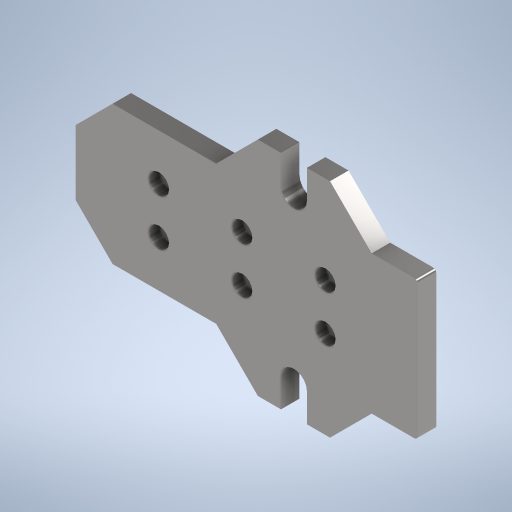
# Autodesk Inventor part: Grundplate
Saved by Autodesk Inventor 2023.2 (Build 272271000, 271)
## iProperties
Created: 2023-02-02
Part Number: Grundplate
Material: Steel, Mild
Document SubType Name: Modeling
Designer: Aditya
Density: 7.85 g/cm^3
Appearance: Semi-Polished
Author: Aditya
Autodesk Inventor part; units mm, degrees
ref_plane "YZ Plane" through (0, 0, 0) normal (1, 0, 0) x (0, 1, 0)
ref_plane "XZ Plane" through (0, 0, 0) normal (0, 1, 0) x (-1, 0, 0)
ref_plane "XY Plane" through (0, 0, 0) normal (0, 0, 1) x (1, 0, 0)
sketch "Sketch1" plane through (0, 0, 0) normal (0, 0, 1) x (1, 0, 0)
  line L0 (92.5, -35.5) -> (92.5, 35.5)
  line L1 (-92.5, 17.5) -> (-92.5, -17.5)
  line L2 (-92.5, 0) -> (-92.5, 17.5)
  line L3 (-92.5, 17.5) -> (-72.5, 37.5)
  line L4 (-92.5, 17.5) -> (-35.0841, 17.5) construction
  line L5 (-92.5, 0) -> (-92.5, -17.5)
  line L6 (-92.5, -17.5) -> (-72.5, -37.5)
  line L7 (25.5, 37.5) -> (25.5, 44.5)
  arc A0 (18.5, 44.5) -> (32.5, 44.5) centre (25.5, 44.5) ccw
  line L8 (32.5, 44.5) -> (32.5, 60)
  line L9 (18.5, 44.5) -> (18.5, 60)
  line L10 (32.5, 60) -> (45, 60)
  line L11 (45, 60) -> (67.5, 37.5)
  line L12 (45, 60) -> (96.9057, 60) construction
  line L13 (18.5, 60) -> (6, 60)
  line L14 (6, 60) -> (-16.5, 37.5)
  line L15 (90.5, 37.5) -> (67.5, 37.5)
  line L16 (-16.5, 37.5) -> (-72.5, 37.5)
  line L17 (25.5, -37.5) -> (25.5, -44.5)
  arc A1 (32.5, -44.5) -> (18.5, -44.5) centre (25.5, -44.5) ccw
  line L18 (18.5, -44.5) -> (18.5, -60)
  line L19 (32.5, -44.5) -> (32.5, -60)
  line L20 (18.5, -60) -> (6, -60)
  line L21 (6, -60) -> (-16.5, -37.5)
  line L22 (32.5, -60) -> (45, -60)
  line L23 (45, -60) -> (67.5, -37.5)
  line L24 (-72.5, -37.5) -> (-16.5, -37.5)
  line L25 (67.5, -37.5) -> (90.5, -37.5)
  arc A2 (92.5, 35.5) -> (90.5, 37.5) centre (90.5, 35.5) ccw
  arc A3 (90.5, -37.5) -> (92.5, -35.5) centre (90.5, -35.5) ccw
  point P0 (0, 0)
  dimension "d13" = 17.5
  dimension "d14" = 45
  dimension "d15" = 17.5
  dimension "d16" = 135
  dimension "d19" = 14
  dimension "d20" = 15.5
  dimension "d21" = 15.5
  dimension "d22" = 12.5
  dimension "d23" = 45
  dimension "d24" = 12.5
  dimension "d25" = 135
  dimension "d27" = 14
  dimension "d28" = 15.5
  dimension "d29" = 15.5
  dimension "d31" = 12.5
  dimension "d32" = 135
  dimension "d33" = 12.5
  dimension "d34" = 135
  dimension "d35" = 2
  dimension "d36" = 60
  dimension "d37" = 185
  dimension "d38" = 97.5
  dimension "d39" = 42.5
  dimension "d40" = 4.4057
  dimension "d41" = 92.5
  dimension "d42" = 60
  dimension "d43" = 127.5841
  constraints: 52 end point, 13 tangent, 10 point on circle, 8 horizontal, 6 parallel, 4 centre point, 4 perpendicular, 4 vertical, 2 coincident, 1 equal radius, 1 midpoint
  measures "d13" distance of L1.start L2.start
  measures "d14" angle of L4 L3
  measures "d15" distance of L1.end L2.start
  measures "d16" angle of L6 L5
  measures "d19" diameter of A0
  measures "d20" distance of L8.start L8.end
  measures "d21" distance of L9.start L9.end
  measures "d22" distance of L8.end L10.end
  measures "d23" angle of L11 L12
  measures "d24" distance of L9.end L13.end
  measures "d25" angle of L14 L13
  measures "d27" diameter of A1
  measures "d28" distance of L18.start L18.end
  measures "d29" distance of L19.start L19.end
  measures "d31" distance of L18.end L20.end
  measures "d32" angle of L20 L21
  measures "d33" distance of L19.end L22.end
  measures "d34" angle of L23 L22
  measures "d35" radius of A2
  measures "d36" distance between parallel lines of L0 L8
  measures "d37" distance between parallel lines of L0 L1
  measures "d38" distance between parallel lines of L12 L25
  measures "d39" distance between parallel lines of L12 L4
  measures "d40" distance from line of L12.end L0
  measures "d41" distance from line of point (0, 0) L0
  measures "d42" distance from line of point (0, 0) L12
  measures "d43" distance from line of L4.end L0
extrude "Extrusion1" add sketch "Sketch1" along normal blind 10
sketch "Sketch2" plane through (0, 0, 10) normal (0, 0, 1) x (1, 0, 0)
  line L0 (92.5, -35.5) -> (92.5, 35.5) projected
  point P0 (0, 0)
  point P1 (42.5, 12.5)
  point P2 (42.5, -12.5)
  point P3 (-2.5, 12.5)
  point P4 (-2.5, -12.5)
  point P5 (-47.5, 12.5)
  point P6 (-47.5, -12.5)
  dimension "d53" = 50
  dimension "d54" = 25
  dimension "d55" = 50
  dimension "d56" = 45
  dimension "d57" = 45
  dimension "d58" = 45
  dimension "d59" = 45
  dimension "d60" = 12.5
  dimension "d61" = 12.5
  dimension "d62" = 12.5
  dimension "d63" = 25
  dimension "d64" = 25
  measures "d53" distance from line of L0 point (42.5, 12.5)
  measures "d54" distance of point (42.5, 12.5) point (42.5, -12.5)
  measures "d55" distance from line of L0 point (42.5, -12.5)
  measures "d56" distance of point (-2.5, 12.5) point (42.5, 12.5)
  measures "d57" distance of point (42.5, -12.5) point (-2.5, -12.5)
  measures "d58" distance of point (-47.5, -12.5) point (-2.5, -12.5)
  measures "d59" distance of point (-2.5, 12.5) point (-47.5, 12.5)
  measures "d60" vertical distance of point (0, 0) point (42.5, -12.5)
  measures "d61" vertical distance of point (-2.5, 12.5) point (0, 0)
  measures "d62" vertical distance of point (0, 0) point (-47.5, 12.5)
  measures "d63" distance of point (-47.5, -12.5) point (-47.5, 12.5)
  measures "d64" distance of point (-2.5, 12.5) point (-2.5, -12.5)
hole "Hole1" at (42.5, 12.5, 10) at (42.5, -12.5, 10) at (-2.5, 12.5, 10) at (-2.5, -12.5, 10) at (-47.5, 12.5, 10) at (-47.5, -12.5, 10) direction (0, 0, -1) diameter 6 end through all counterbore diameter 11 counterbore depth 6
body "Solid1"
